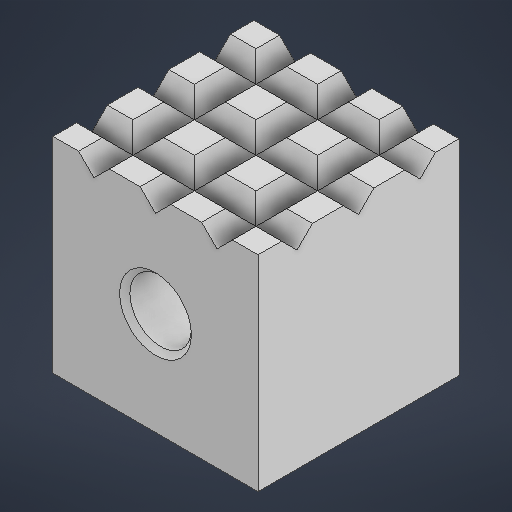
# Autodesk Inventor part: Foot
Saved by Autodesk Inventor 2025.4 (Build 294407000, 407)
## iProperties
Created: 2026-05-27
Part Number: Foot
Material: Generic
Document SubType Name: Modeling
Designer: VuQuan
Density: 1 g/cm^3
Appearance: Default
Author: VuQuan
Autodesk Inventor part; units mm, degrees
ref_plane "YZ Plane" through (0, 0, 0) normal (1, 0, 0) x (0, 1, 0)
ref_plane "XZ Plane" through (0, 0, 0) normal (0, 1, 0) x (-1, 0, 0)
ref_plane "XY Plane" through (0, 0, 0) normal (0, 0, 1) x (1, 0, 0)
sketch "Sketch1" plane through (0, 0, 0) normal (0, 0, 1) x (1, 0, 0)
  line L0 (-10, 0) -> (0, 0)
  line L1 (-10, 0) -> (-10, 20)
  line L2 (-10, 20) -> (-7.5, 20)
  line L3 (-4.5, 20) -> (-1.5, 20)
  line L4 (-7.5, 20) -> (-6, 18.5)
  line L5 (-6, 18.5) -> (-4.5, 20)
  line L6 (-1.5, 20) -> (0, 18.5)
  line L7 (0, 18.5) -> (0, 0) construction
  line L8 (10, 0) -> (0, 0)
  line L9 (10, 0) -> (10, 20)
  line L10 (10, 20) -> (7.5, 20)
  line L11 (4.5, 20) -> (1.5, 20)
  line L12 (7.5, 20) -> (6, 18.5)
  line L13 (6, 18.5) -> (4.5, 20)
  line L14 (1.5, 20) -> (0, 18.5)
  circle A0 centre (0, 10) radius 3
  dimension "d0" = 6
  dimension "d1" = 20
  dimension "d2" = 20
  dimension "d3" = 1.5
  dimension "d4" = 6
  dimension "d5" = 10
  constraints: 32 end point, 6 symmetric about line, 5 point on line, 2 coincident, 2 equal length, 2 perpendicular, 2 vertical, 1 centre point, 1 horizontal, 1 horizontal alignment
  measures "d0" distance of L6.end L4.end
  measures "d1" distance between parallel lines of L0 L2
  measures "d2" diameter of L1 L7
  measures "d3" distance from line of L2 L4.end
  measures "d4" diameter of A0
  measures "d5" distance from line of L0 A0.centre
extrude "Extrusion1" add sketch "Sketch1" along normal mid plane 19.6
sketch "Sketch2" plane through (10, 0, 9.8) normal (1, 0, 0) x (0, 0, -1)
  line L0 (19.6, 20) -> (0, 20) projected
  line L1 (9.8, 20) -> (9.8, 0) construction
  line L2 (0, 13) -> (19.6, 13) projected
  line L3 (2.3, 20) -> (3.8, 18.5)
  line L4 (3.8, 18.5) -> (5.3, 20)
  line L5 (19.6, 20) -> (0, 20) projected
  line L6 (8.3, 20) -> (9.8, 18.5)
  line L7 (17.3, 20) -> (15.8, 18.5)
  line L8 (15.8, 18.5) -> (14.3, 20)
  line L9 (11.3, 20) -> (9.8, 18.5)
  dimension "d8" = 1.5
  dimension "d9" = 6
  constraints: 14 end point, 4 point on line, 4 symmetric about line, 3 perpendicular, 1 horizontal alignment, 1 midpoint, 1 parallel
  measures "d8" distance from line of L0 L3.end
  measures "d9" distance from line of L3.end L1
extrude "Extrusion2" cut sketch "Sketch2" against normal through all
chamfer "Chamfer1" distance 0.5 angle 45 1 edges at (-3, 10, 9.8)
body "Solid1"
